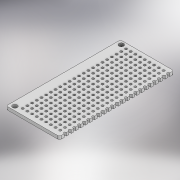
# Autodesk Inventor part: Modulo MPU 6050
Saved by Autodesk Inventor 2021.4 (Build 254397000, 397)
## iProperties
Created: 2022-11-18
Part Number: Modulo MPU 6050
Material: Genérico
Document SubType Name: Modeling
Designer: crist
Density: 1 g/cm^3
Appearance: Valor por defecto
Author: crist
Autodesk Inventor part; units mm, degrees
ref_plane "YZ Plane" through (0, 0, 0) normal (1, 0, 0) x (0, 1, 0)
ref_plane "XZ Plane" through (0, 0, 0) normal (0, 1, 0) x (-1, 0, 0)
ref_plane "XY Plane" through (0, 0, 0) normal (0, 0, 1) x (1, 0, 0)
sketch "Boceto1" plane through (0, 0, 0) normal (0, 1, 0) x (-1, 0, 0)
  line L0 (1, 0) -> (33, 0)
  line L1 (34, -1) -> (34, -72)
  line L2 (33, -73) -> (1, -73)
  line L3 (0, -72) -> (0, -1)
  arc A0 (34, -1) -> (33, 0) centre (33, -1) ccw
  arc A1 (1, 0) -> (0, -1) centre (1, -1) ccw
  arc A2 (0, -72) -> (1, -73) centre (1, -72) ccw
  arc A3 (33, -73) -> (34, -72) centre (33, -72) ccw
  line L4 (34, -73) -> (33, -73)
  line L5 (33, -73) -> (32.5, -73)
  line L6 (32.5, -73) -> (32.5, -72)
  line L7 (32.5, -72) -> (31, -72)
  line L8 (31, -72) -> (31, -70.5)
  circle A4 centre (31, -70.5) radius 1.5
  line L9 (34, -36.5) -> (7.9198, -36.5)
  circle A5 centre (31, -2.5) radius 1.5
  point P0 (0, 0)
  point P1 (34, 0)
  point P2 (0, -73)
  dimension "d0" = 34
  dimension "d1" = 73
  dimension "d2" = 1
  dimension "d5" = 1
  dimension "d6" = 0.5
  dimension "d7" = 1
  dimension "d8" = 1.5
  dimension "d9" = 1.5
  constraints: 20 end point, 9 point on line, 9 tangent, 8 point on circle, 5 centre point, 3 equal radius, 3 horizontal, 3 perpendicular, 2 parallel, 1 coincident, 1 collinear, 1 midpoint, 1 symmetric about line, 1 vertical alignment, 3 other
  measures "d0" distance of L4.start point (0, -73)
  measures "d1" distance of point (34, 0) L4.start
  measures "d2" radius of A0
  measures "d5" distance of L4.start L2.start
  measures "d6" distance of L2.start L5.end
  measures "d7" distance of L5.end L6.end
  measures "d8" distance of L6.end L7.end
  measures "d9" distance of L7.end L8.end
extrude "Extrusión1" add sketch "Boceto1" along normal blind 2
sketch "Boceto2" plane through (0, 2, 0) normal (0, 1, 0) x (1, 0, 0)
  line L0 (-34, 72) -> (-34, 1) projected
  line L1 (-34, 73) -> (-28, 73)
  line L2 (-1, 73) -> (-33, 73) projected
  line L3 (-28, 73) -> (-28, 70.5)
  line L4 (-28, 70.5) -> (-27.25, 70.5)
  line L5 (-27.25, 70.5) -> (-27.25, 69.75)
  circle A0 centre (-27.25, 69.75) radius 0.75
  circle A1 centre (-24.25, 69.75) radius 0.75
  circle A2 centre (-21.25, 69.75) radius 0.75
  circle A3 centre (-18.25, 69.75) radius 0.75
  circle A4 centre (-15.25, 69.75) radius 0.75
  circle A5 centre (-12.25, 69.75) radius 0.75
  circle A6 centre (-9.25, 69.75) radius 0.75
  circle A7 centre (-6.25, 69.75) radius 0.75
  circle A8 centre (-3.25, 69.75) radius 0.75
  circle A9 centre (-0.25, 69.75) radius 0.75
  circle A10 centre (-27.25, 66.75) radius 0.75
  circle A11 centre (-24.25, 66.75) radius 0.75
  circle A12 centre (-21.25, 66.75) radius 0.75
  circle A13 centre (-18.25, 66.75) radius 0.75
  circle A14 centre (-15.25, 66.75) radius 0.75
  circle A15 centre (-12.25, 66.75) radius 0.75
  circle A16 centre (-9.25, 66.75) radius 0.75
  circle A17 centre (-6.25, 66.75) radius 0.75
  circle A18 centre (-3.25, 66.75) radius 0.75
  circle A19 centre (-0.25, 66.75) radius 0.75
  circle A20 centre (-27.25, 63.75) radius 0.75
  circle A21 centre (-24.25, 63.75) radius 0.75
  circle A22 centre (-21.25, 63.75) radius 0.75
  circle A23 centre (-18.25, 63.75) radius 0.75
  circle A24 centre (-15.25, 63.75) radius 0.75
  circle A25 centre (-12.25, 63.75) radius 0.75
  circle A26 centre (-9.25, 63.75) radius 0.75
  circle A27 centre (-6.25, 63.75) radius 0.75
  circle A28 centre (-3.25, 63.75) radius 0.75
  circle A29 centre (-0.25, 63.75) radius 0.75
  circle A30 centre (-27.25, 60.75) radius 0.75
  circle A31 centre (-24.25, 60.75) radius 0.75
  circle A32 centre (-21.25, 60.75) radius 0.75
  circle A33 centre (-18.25, 60.75) radius 0.75
  circle A34 centre (-15.25, 60.75) radius 0.75
  circle A35 centre (-12.25, 60.75) radius 0.75
  circle A36 centre (-9.25, 60.75) radius 0.75
  circle A37 centre (-6.25, 60.75) radius 0.75
  circle A38 centre (-3.25, 60.75) radius 0.75
  circle A39 centre (-0.25, 60.75) radius 0.75
  circle A40 centre (-27.25, 57.75) radius 0.75
  circle A41 centre (-24.25, 57.75) radius 0.75
  circle A42 centre (-21.25, 57.75) radius 0.75
  circle A43 centre (-18.25, 57.75) radius 0.75
  circle A44 centre (-15.25, 57.75) radius 0.75
  circle A45 centre (-12.25, 57.75) radius 0.75
  circle A46 centre (-9.25, 57.75) radius 0.75
  circle A47 centre (-6.25, 57.75) radius 0.75
  circle A48 centre (-3.25, 57.75) radius 0.75
  circle A49 centre (-0.25, 57.75) radius 0.75
  circle A50 centre (-27.25, 54.75) radius 0.75
  circle A51 centre (-24.25, 54.75) radius 0.75
  circle A52 centre (-21.25, 54.75) radius 0.75
  circle A53 centre (-18.25, 54.75) radius 0.75
  circle A54 centre (-15.25, 54.75) radius 0.75
  circle A55 centre (-12.25, 54.75) radius 0.75
  circle A56 centre (-9.25, 54.75) radius 0.75
  circle A57 centre (-6.25, 54.75) radius 0.75
  circle A58 centre (-3.25, 54.75) radius 0.75
  circle A59 centre (-0.25, 54.75) radius 0.75
  circle A60 centre (-27.25, 51.75) radius 0.75
  circle A61 centre (-24.25, 51.75) radius 0.75
  circle A62 centre (-21.25, 51.75) radius 0.75
  circle A63 centre (-18.25, 51.75) radius 0.75
  circle A64 centre (-15.25, 51.75) radius 0.75
  circle A65 centre (-12.25, 51.75) radius 0.75
  circle A66 centre (-9.25, 51.75) radius 0.75
  circle A67 centre (-6.25, 51.75) radius 0.75
  circle A68 centre (-3.25, 51.75) radius 0.75
  circle A69 centre (-0.25, 51.75) radius 0.75
  circle A70 centre (-27.25, 48.75) radius 0.75
  circle A71 centre (-24.25, 48.75) radius 0.75
  circle A72 centre (-21.25, 48.75) radius 0.75
  circle A73 centre (-18.25, 48.75) radius 0.75
  circle A74 centre (-15.25, 48.75) radius 0.75
  circle A75 centre (-12.25, 48.75) radius 0.75
  circle A76 centre (-9.25, 48.75) radius 0.75
  circle A77 centre (-6.25, 48.75) radius 0.75
  circle A78 centre (-3.25, 48.75) radius 0.75
  circle A79 centre (-0.25, 48.75) radius 0.75
  circle A80 centre (-27.25, 45.75) radius 0.75
  circle A81 centre (-24.25, 45.75) radius 0.75
  circle A82 centre (-21.25, 45.75) radius 0.75
  circle A83 centre (-18.25, 45.75) radius 0.75
  circle A84 centre (-15.25, 45.75) radius 0.75
  circle A85 centre (-12.25, 45.75) radius 0.75
  circle A86 centre (-9.25, 45.75) radius 0.75
  circle A87 centre (-6.25, 45.75) radius 0.75
  circle A88 centre (-3.25, 45.75) radius 0.75
  circle A89 centre (-0.25, 45.75) radius 0.75
  circle A90 centre (-27.25, 42.75) radius 0.75
  circle A91 centre (-24.25, 42.75) radius 0.75
  circle A92 centre (-21.25, 42.75) radius 0.75
  circle A93 centre (-18.25, 42.75) radius 0.75
  circle A94 centre (-15.25, 42.75) radius 0.75
  circle A95 centre (-12.25, 42.75) radius 0.75
  circle A96 centre (-9.25, 42.75) radius 0.75
  circle A97 centre (-6.25, 42.75) radius 0.75
  circle A98 centre (-3.25, 42.75) radius 0.75
  circle A99 centre (-0.25, 42.75) radius 0.75
  circle A100 centre (-27.25, 39.75) radius 0.75
  circle A101 centre (-24.25, 39.75) radius 0.75
  circle A102 centre (-21.25, 39.75) radius 0.75
  circle A103 centre (-18.25, 39.75) radius 0.75
  circle A104 centre (-15.25, 39.75) radius 0.75
  circle A105 centre (-12.25, 39.75) radius 0.75
  circle A106 centre (-9.25, 39.75) radius 0.75
  circle A107 centre (-6.25, 39.75) radius 0.75
  circle A108 centre (-3.25, 39.75) radius 0.75
  circle A109 centre (-0.25, 39.75) radius 0.75
  circle A110 centre (-27.25, 36.75) radius 0.75
  circle A111 centre (-24.25, 36.75) radius 0.75
  circle A112 centre (-21.25, 36.75) radius 0.75
  circle A113 centre (-18.25, 36.75) radius 0.75
  circle A114 centre (-15.25, 36.75) radius 0.75
  circle A115 centre (-12.25, 36.75) radius 0.75
  circle A116 centre (-9.25, 36.75) radius 0.75
  circle A117 centre (-6.25, 36.75) radius 0.75
  circle A118 centre (-3.25, 36.75) radius 0.75
  circle A119 centre (-0.25, 36.75) radius 0.75
  circle A120 centre (-27.25, 33.75) radius 0.75
  circle A121 centre (-24.25, 33.75) radius 0.75
  circle A122 centre (-21.25, 33.75) radius 0.75
  circle A123 centre (-18.25, 33.75) radius 0.75
  circle A124 centre (-15.25, 33.75) radius 0.75
  circle A125 centre (-12.25, 33.75) radius 0.75
  circle A126 centre (-9.25, 33.75) radius 0.75
  circle A127 centre (-6.25, 33.75) radius 0.75
  circle A128 centre (-3.25, 33.75) radius 0.75
  circle A129 centre (-0.25, 33.75) radius 0.75
  circle A130 centre (-27.25, 30.75) radius 0.75
  circle A131 centre (-24.25, 30.75) radius 0.75
  circle A132 centre (-21.25, 30.75) radius 0.75
  circle A133 centre (-18.25, 30.75) radius 0.75
  circle A134 centre (-15.25, 30.75) radius 0.75
  circle A135 centre (-12.25, 30.75) radius 0.75
  circle A136 centre (-9.25, 30.75) radius 0.75
  circle A137 centre (-6.25, 30.75) radius 0.75
  circle A138 centre (-3.25, 30.75) radius 0.75
  circle A139 centre (-0.25, 30.75) radius 0.75
  circle A140 centre (-27.25, 27.75) radius 0.75
  circle A141 centre (-24.25, 27.75) radius 0.75
  circle A142 centre (-21.25, 27.75) radius 0.75
  circle A143 centre (-18.25, 27.75) radius 0.75
  circle A144 centre (-15.25, 27.75) radius 0.75
  circle A145 centre (-12.25, 27.75) radius 0.75
  circle A146 centre (-9.25, 27.75) radius 0.75
  circle A147 centre (-6.25, 27.75) radius 0.75
  circle A148 centre (-3.25, 27.75) radius 0.75
  circle A149 centre (-0.25, 27.75) radius 0.75
  circle A150 centre (-27.25, 24.75) radius 0.75
  circle A151 centre (-24.25, 24.75) radius 0.75
  circle A152 centre (-21.25, 24.75) radius 0.75
  circle A153 centre (-18.25, 24.75) radius 0.75
  circle A154 centre (-15.25, 24.75) radius 0.75
  circle A155 centre (-12.25, 24.75) radius 0.75
  circle A156 centre (-9.25, 24.75) radius 0.75
  circle A157 centre (-6.25, 24.75) radius 0.75
  circle A158 centre (-3.25, 24.75) radius 0.75
  circle A159 centre (-0.25, 24.75) radius 0.75
  circle A160 centre (-27.25, 21.75) radius 0.75
  circle A161 centre (-24.25, 21.75) radius 0.75
  circle A162 centre (-21.25, 21.75) radius 0.75
  circle A163 centre (-18.25, 21.75) radius 0.75
  circle A164 centre (-15.25, 21.75) radius 0.75
  circle A165 centre (-12.25, 21.75) radius 0.75
  circle A166 centre (-9.25, 21.75) radius 0.75
  circle A167 centre (-6.25, 21.75) radius 0.75
  circle A168 centre (-3.25, 21.75) radius 0.75
  circle A169 centre (-0.25, 21.75) radius 0.75
  circle A170 centre (-27.25, 18.75) radius 0.75
  circle A171 centre (-24.25, 18.75) radius 0.75
  circle A172 centre (-21.25, 18.75) radius 0.75
  circle A173 centre (-18.25, 18.75) radius 0.75
  circle A174 centre (-15.25, 18.75) radius 0.75
  circle A175 centre (-12.25, 18.75) radius 0.75
  circle A176 centre (-9.25, 18.75) radius 0.75
  circle A177 centre (-6.25, 18.75) radius 0.75
  circle A178 centre (-3.25, 18.75) radius 0.75
  circle A179 centre (-0.25, 18.75) radius 0.75
  circle A180 centre (-27.25, 15.75) radius 0.75
  circle A181 centre (-24.25, 15.75) radius 0.75
  circle A182 centre (-21.25, 15.75) radius 0.75
  circle A183 centre (-18.25, 15.75) radius 0.75
  circle A184 centre (-15.25, 15.75) radius 0.75
  circle A185 centre (-12.25, 15.75) radius 0.75
  circle A186 centre (-9.25, 15.75) radius 0.75
  circle A187 centre (-6.25, 15.75) radius 0.75
  circle A188 centre (-3.25, 15.75) radius 0.75
  circle A189 centre (-0.25, 15.75) radius 0.75
  circle A190 centre (-27.25, 12.75) radius 0.75
  circle A191 centre (-24.25, 12.75) radius 0.75
  circle A192 centre (-21.25, 12.75) radius 0.75
  circle A193 centre (-18.25, 12.75) radius 0.75
  circle A194 centre (-15.25, 12.75) radius 0.75
  circle A195 centre (-12.25, 12.75) radius 0.75
  circle A196 centre (-9.25, 12.75) radius 0.75
  circle A197 centre (-6.25, 12.75) radius 0.75
  circle A198 centre (-3.25, 12.75) radius 0.75
  circle A199 centre (-0.25, 12.75) radius 0.75
  circle A200 centre (-27.25, 9.75) radius 0.75
  circle A201 centre (-24.25, 9.75) radius 0.75
  circle A202 centre (-21.25, 9.75) radius 0.75
  circle A203 centre (-18.25, 9.75) radius 0.75
  circle A204 centre (-15.25, 9.75) radius 0.75
  circle A205 centre (-12.25, 9.75) radius 0.75
  circle A206 centre (-9.25, 9.75) radius 0.75
  circle A207 centre (-6.25, 9.75) radius 0.75
  circle A208 centre (-3.25, 9.75) radius 0.75
  circle A209 centre (-0.25, 9.75) radius 0.75
  circle A210 centre (-27.25, 6.75) radius 0.75
  circle A211 centre (-24.25, 6.75) radius 0.75
  circle A212 centre (-21.25, 6.75) radius 0.75
  circle A213 centre (-18.25, 6.75) radius 0.75
  circle A214 centre (-15.25, 6.75) radius 0.75
  circle A215 centre (-12.25, 6.75) radius 0.75
  circle A216 centre (-9.25, 6.75) radius 0.75
  circle A217 centre (-6.25, 6.75) radius 0.75
  circle A218 centre (-3.25, 6.75) radius 0.75
  circle A219 centre (-0.25, 6.75) radius 0.75
  circle A220 centre (-27.25, 3.75) radius 0.75
  circle A221 centre (-24.25, 3.75) radius 0.75
  circle A222 centre (-21.25, 3.75) radius 0.75
  circle A223 centre (-18.25, 3.75) radius 0.75
  circle A224 centre (-15.25, 3.75) radius 0.75
  circle A225 centre (-12.25, 3.75) radius 0.75
  circle A226 centre (-9.25, 3.75) radius 0.75
  circle A227 centre (-6.25, 3.75) radius 0.75
  circle A228 centre (-3.25, 3.75) radius 0.75
  circle A229 centre (-0.25, 3.75) radius 0.75
  point P0 (0, 0)
  point P1 (-24.25, 70.5)
  point P2 (-21.25, 70.5)
  point P3 (-18.25, 70.5)
  point P4 (-15.25, 70.5)
  point P5 (-12.25, 70.5)
  point P6 (-9.25, 70.5)
  point P7 (-6.25, 70.5)
  point P8 (-3.25, 70.5)
  point P9 (-0.25, 70.5)
  point P10 (-27.25, 67.5)
  point P11 (-24.25, 67.5)
  point P12 (-21.25, 67.5)
  point P13 (-18.25, 67.5)
  point P14 (-15.25, 67.5)
  point P15 (-12.25, 67.5)
  point P16 (-9.25, 67.5)
  point P17 (-6.25, 67.5)
  point P18 (-3.25, 67.5)
  point P19 (-0.25, 67.5)
  point P20 (-27.25, 64.5)
  point P21 (-24.25, 64.5)
  point P22 (-21.25, 64.5)
  point P23 (-18.25, 64.5)
  point P24 (-15.25, 64.5)
  point P25 (-12.25, 64.5)
  point P26 (-9.25, 64.5)
  point P27 (-6.25, 64.5)
  point P28 (-3.25, 64.5)
  point P29 (-0.25, 64.5)
  point P30 (-27.25, 61.5)
  point P31 (-24.25, 61.5)
  point P32 (-21.25, 61.5)
  point P33 (-18.25, 61.5)
  point P34 (-15.25, 61.5)
  point P35 (-12.25, 61.5)
  point P36 (-9.25, 61.5)
  point P37 (-6.25, 61.5)
  point P38 (-3.25, 61.5)
  point P39 (-0.25, 61.5)
  point P40 (-27.25, 58.5)
  point P41 (-24.25, 58.5)
  point P42 (-21.25, 58.5)
  point P43 (-18.25, 58.5)
  point P44 (-15.25, 58.5)
  point P45 (-12.25, 58.5)
  point P46 (-9.25, 58.5)
  point P47 (-6.25, 58.5)
  point P48 (-3.25, 58.5)
  point P49 (-0.25, 58.5)
  point P50 (-27.25, 55.5)
  point P51 (-24.25, 55.5)
  point P52 (-21.25, 55.5)
  point P53 (-18.25, 55.5)
  point P54 (-15.25, 55.5)
  point P55 (-12.25, 55.5)
  point P56 (-9.25, 55.5)
  point P57 (-6.25, 55.5)
  point P58 (-3.25, 55.5)
  point P59 (-0.25, 55.5)
  point P60 (-27.25, 52.5)
  point P61 (-24.25, 52.5)
  point P62 (-21.25, 52.5)
  point P63 (-18.25, 52.5)
  point P64 (-15.25, 52.5)
  point P65 (-12.25, 52.5)
  point P66 (-9.25, 52.5)
  point P67 (-6.25, 52.5)
  point P68 (-3.25, 52.5)
  point P69 (-0.25, 52.5)
  point P70 (-27.25, 49.5)
  point P71 (-24.25, 49.5)
  point P72 (-21.25, 49.5)
  point P73 (-18.25, 49.5)
  point P74 (-15.25, 49.5)
  point P75 (-12.25, 49.5)
  point P76 (-9.25, 49.5)
  point P77 (-6.25, 49.5)
  point P78 (-3.25, 49.5)
  point P79 (-0.25, 49.5)
  point P80 (-27.25, 46.5)
  point P81 (-24.25, 46.5)
  point P82 (-21.25, 46.5)
  point P83 (-18.25, 46.5)
  point P84 (-15.25, 46.5)
  point P85 (-12.25, 46.5)
  point P86 (-9.25, 46.5)
  point P87 (-6.25, 46.5)
  point P88 (-3.25, 46.5)
  point P89 (-0.25, 46.5)
  point P90 (-27.25, 43.5)
  point P91 (-24.25, 43.5)
  point P92 (-21.25, 43.5)
  point P93 (-18.25, 43.5)
  point P94 (-15.25, 43.5)
  point P95 (-12.25, 43.5)
  point P96 (-9.25, 43.5)
  point P97 (-6.25, 43.5)
  point P98 (-3.25, 43.5)
  point P99 (-0.25, 43.5)
  point P100 (-27.25, 40.5)
  point P101 (-24.25, 40.5)
  point P102 (-21.25, 40.5)
  point P103 (-18.25, 40.5)
  point P104 (-15.25, 40.5)
  point P105 (-12.25, 40.5)
  point P106 (-9.25, 40.5)
  point P107 (-6.25, 40.5)
  point P108 (-3.25, 40.5)
  point P109 (-0.25, 40.5)
  point P110 (-27.25, 37.5)
  point P111 (-24.25, 37.5)
  point P112 (-21.25, 37.5)
  point P113 (-18.25, 37.5)
  point P114 (-15.25, 37.5)
  point P115 (-12.25, 37.5)
  point P116 (-9.25, 37.5)
  point P117 (-6.25, 37.5)
  point P118 (-3.25, 37.5)
  point P119 (-0.25, 37.5)
  point P120 (-27.25, 34.5)
  point P121 (-24.25, 34.5)
  point P122 (-21.25, 34.5)
  point P123 (-18.25, 34.5)
  point P124 (-15.25, 34.5)
  point P125 (-12.25, 34.5)
  point P126 (-9.25, 34.5)
  point P127 (-6.25, 34.5)
  point P128 (-3.25, 34.5)
  point P129 (-0.25, 34.5)
  point P130 (-27.25, 31.5)
  point P131 (-24.25, 31.5)
  point P132 (-21.25, 31.5)
  point P133 (-18.25, 31.5)
  point P134 (-15.25, 31.5)
  point P135 (-12.25, 31.5)
  point P136 (-9.25, 31.5)
  point P137 (-6.25, 31.5)
  point P138 (-3.25, 31.5)
  point P139 (-0.25, 31.5)
  point P140 (-27.25, 28.5)
  point P141 (-24.25, 28.5)
  point P142 (-21.25, 28.5)
  point P143 (-18.25, 28.5)
  point P144 (-15.25, 28.5)
  point P145 (-12.25, 28.5)
  point P146 (-9.25, 28.5)
  point P147 (-6.25, 28.5)
  point P148 (-3.25, 28.5)
  point P149 (-0.25, 28.5)
  point P150 (-27.25, 25.5)
  point P151 (-24.25, 25.5)
  point P152 (-21.25, 25.5)
  point P153 (-18.25, 25.5)
  point P154 (-15.25, 25.5)
  point P155 (-12.25, 25.5)
  point P156 (-9.25, 25.5)
  point P157 (-6.25, 25.5)
  point P158 (-3.25, 25.5)
  point P159 (-0.25, 25.5)
  point P160 (-27.25, 22.5)
  point P161 (-24.25, 22.5)
  point P162 (-21.25, 22.5)
  point P163 (-18.25, 22.5)
  point P164 (-15.25, 22.5)
  point P165 (-12.25, 22.5)
  point P166 (-9.25, 22.5)
  point P167 (-6.25, 22.5)
  point P168 (-3.25, 22.5)
  point P169 (-0.25, 22.5)
  point P170 (-27.25, 19.5)
  point P171 (-24.25, 19.5)
  point P172 (-21.25, 19.5)
  point P173 (-18.25, 19.5)
  point P174 (-15.25, 19.5)
  point P175 (-12.25, 19.5)
  point P176 (-9.25, 19.5)
  point P177 (-6.25, 19.5)
  point P178 (-3.25, 19.5)
  point P179 (-0.25, 19.5)
  point P180 (-27.25, 16.5)
  point P181 (-24.25, 16.5)
  point P182 (-21.25, 16.5)
  point P183 (-18.25, 16.5)
  point P184 (-15.25, 16.5)
  point P185 (-12.25, 16.5)
  point P186 (-9.25, 16.5)
  point P187 (-6.25, 16.5)
  point P188 (-3.25, 16.5)
  point P189 (-0.25, 16.5)
  point P190 (-27.25, 13.5)
  point P191 (-24.25, 13.5)
  point P192 (-21.25, 13.5)
  point P193 (-18.25, 13.5)
  point P194 (-15.25, 13.5)
  point P195 (-12.25, 13.5)
  point P196 (-9.25, 13.5)
  point P197 (-6.25, 13.5)
  point P198 (-3.25, 13.5)
  point P199 (-0.25, 13.5)
  dimension "d12" = 6
  dimension "d13" = 2.5
  dimension "d14" = 0.75
  dimension "d18" = 3
  dimension "d21" = 3
  constraints: 230 vertical alignment, 221 vertical, 11 horizontal, 8 end point, 1 coincident, 1 perpendicular, 1 point on line, 918 other
  measures "d12" distance of L1.start L1.end
  measures "d13" distance of L1.end L3.end
  measures "d14" distance of L3.end L4.end
  measures "d18" distance of point (-27.25, 69.75) point (-24.25, 69.75)
  measures "d21" distance of point (-27.25, 69.75) point (-27.25, 66.75)
extrude "Extrusión2" cut sketch "Boceto2" against normal blind 3
